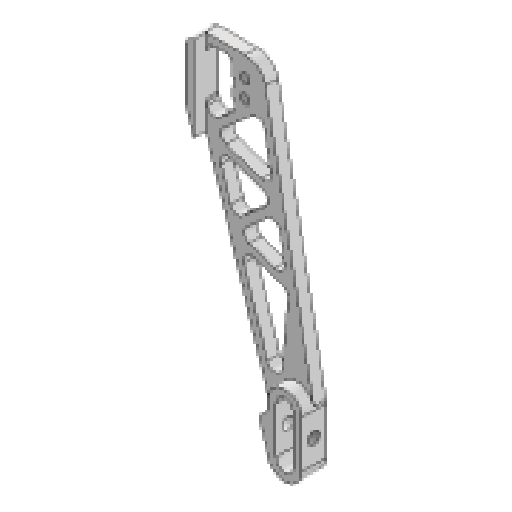
# Autodesk Inventor part: VerticalSlideMiddleTop2.2
Saved by Autodesk Inventor 2023 (Build 270158000, 158)
## iProperties
Created: 2022-10-14
Part Number: VerticalSlideMiddleTop2.2
Material: Generic
Document SubType Name: Modeling
Designer: deli
Density: 1 g/cm^3
Appearance: Default
Mass: 2.31146 g
Surface Area: 29.6295 cm^2
Volume: 2.31146 cm^3
Author: deli
Autodesk Inventor part; units mm, degrees
ref_plane "YZ Plane" through (0, 0, 0) normal (1, 0, 0) x (0, 1, 0)
ref_plane "XZ Plane" through (0, 0, 0) normal (0, 1, 0) x (-1, 0, 0)
ref_plane "XY Plane" through (0, 0, 0) normal (0, 0, 1) x (1, 0, 0)
sketch "Sketch1" plane through (0, 0, 0) normal (0, 0, 1) x (1, 0, 0)
  line L0 (-75.161949, -110.524663) -> (-75.161949, -123.524663)
  line L1 (-75.07064, -124.122072) -> (-53.967918, -191.544158)
  circle A0 centre (-63.161949, -118.274663) radius 1.25
  circle A1 centre (-63.161949, -113.774663) radius 1.25
  arc A2 (-52.161949, -190.274663) -> (-47.661949, -190.274663) centre (-49.911949, -190.274663) ccw
  arc A3 (-47.661949, -178.274663) -> (-52.161949, -178.274663) centre (-49.911949, -178.274663) ccw
  line L2 (-47.661949, -178.274663) -> (-47.661949, -190.274663)
  line L3 (-52.161949, -178.274663) -> (-52.161949, -190.274663)
  line L4 (-45.661949, -178.274663) -> (-45.661949, -190.274663)
  arc A4 (-53.967918, -191.544158) -> (-45.661949, -190.274663) centre (-49.911949, -190.274663) ccw
  arc A5 (-45.661949, -178.274663) -> (-45.736374, -177.482781) centre (-49.911949, -178.274663) ccw
  line L5 (-45.736374, -177.482781) -> (-58.003886, -112.796456)
  line L6 (-73.161949, -108.524663) -> (-63.161949, -108.524663)
  arc A6 (-58.003886, -112.796456) -> (-63.161949, -108.524663) centre (-63.161949, -113.774663) ccw
  arc A7 (-73.161949, -108.524663) -> (-75.161949, -110.524663) centre (-73.161949, -110.524663) ccw
  arc A8 (-75.161949, -123.524663) -> (-75.07064, -124.122072) centre (-73.161949, -123.524663) ccw
  line L7 (-52.161949, -182.774663) -> (-56.161949, -182.774663)
  line L8 (-56.161949, -182.774663) -> (-56.161949, -185.774663)
  line L9 (-56.161949, -185.774663) -> (-52.161949, -185.774663)
  point P0 (0, 0)
  dimension "d2" = 2.5
  dimension "d11" = 2
  dimension "d22" = 12
  dimension "d46" = 2
  dimension "d47" = 4.5
  dimension "d84" = 4
  dimension "d86" = 12
  dimension "d87" = 12
  dimension "d88" = 23
  dimension "d90" = 4
  dimension "d91" = 3
  dimension "d92" = 4.5
  dimension "d94" = 15
  dimension "d96" = 2
  dimension "d147" = 72
  constraints: 20 end point, 16 point on circle, 13 tangent, 9 centre point, 4 equal radius, 4 point on line, 3 perpendicular, 2 coincident, 2 vertical, 1 concentric, 1 horizontal, 1 parallel
  measures "d2" diameter of A0
  measures "d22" distance of A2.centre A3.centre
  measures "d46" radial gap between concentric circles of A4 A2
  measures "d47" distance between parallel lines of L2 L3
  measures "d84" distance edge to line of A1 L6
  measures "d86" distance from line of A1.centre L0
  measures "d87" distance from line of A0.centre L0
  measures "d88" distance between parallel lines of L3 L0
  measures "d90" distance of L7.start L7.end
  measures "d91" distance of L7.end L8.end
  measures "d92" distance from line of L3.start L7
  measures "d94" distance from line of L6 L0.end
  measures "d96" radius of A7
  measures "d147" vertical distance of A2.centre A0.centre
extrude "Extrusion1" add sketch "Sketch1" along normal blind 6.35 contours A7 L6 A6 L5 A5 L4 A4 L1 L9 L3 A2 L2 A3 L7 L8 A8 L0 | L8 L7 L3 L9 L1
thread "Thread2" size "M3x0.5" class "6H" standard "ANSI Metric M Profile" full length
thread "Thread6" size "M3x0.5" class "6H" standard "ANSI Metric M Profile" full length
sketch "Sketch12" plane through (0, 0, 6.35) normal (0, 0, 1) x (1, 0, 0)
  line L0 (-75.161949, -110.524663) -> (-75.161949, -123.524663)
  arc A0 (-75.161949, -123.524663) -> (-75.07064, -124.122072) centre (-73.161949, -123.524663) ccw
  line L1 (-75.07064, -124.122072) -> (-53.967918, -191.544158)
  arc A1 (-53.967918, -191.544158) -> (-45.661949, -190.274663) centre (-49.911949, -190.274663) ccw
  line L2 (-45.661949, -190.274663) -> (-45.661949, -178.274663)
  arc A2 (-45.661949, -178.274663) -> (-45.736374, -177.482781) centre (-49.911949, -178.274663) ccw
  line L3 (-45.736374, -177.482781) -> (-58.003886, -112.796456)
  arc A3 (-58.003886, -112.796456) -> (-63.161949, -108.524663) centre (-63.161949, -113.774663) ccw
  line L4 (-63.161949, -108.524663) -> (-73.161949, -108.524663)
  arc A4 (-73.161949, -108.524663) -> (-75.161949, -110.524663) centre (-73.161949, -110.524663) ccw
  circle A5 centre (-63.161949, -118.274663) radius 1.25
  circle A6 centre (-63.161949, -113.774663) radius 1.25
  line L5 (-47.661949, -178.274663) -> (-47.661949, -190.274663)
  arc A7 (-52.161949, -190.274663) -> (-47.661949, -190.274663) centre (-49.911949, -190.274663) ccw
  line L6 (-52.161949, -190.274663) -> (-52.161949, -178.274663)
  arc A8 (-47.661949, -178.274663) -> (-52.161949, -178.274663) centre (-49.911949, -178.274663) ccw
  line L7 (-73.161949, -123.524663) -> (-73.161949, -110.524663)
  line L8 (-73.161949, -110.524663) -> (-63.161949, -110.524663)
  line L9 (-59.968862, -113.169106) -> (-48.373155, -174.31302)
  line L10 (-54.161949, -184.228661) -> (-73.161949, -123.524663)
  line L11 (-54.161949, -178.274663) -> (-54.161949, -184.228661)
  arc A9 (-65.507157, -116.024663) -> (-60.816741, -116.024663) centre (-63.161949, -118.274663) ccw
  arc A10 (-63.161949, -110.524663) -> (-65.507157, -116.024663) centre (-63.161949, -113.774663) ccw
  arc A11 (-60.816741, -116.024663) -> (-59.968862, -113.169106) centre (-63.161949, -113.774663) ccw
  arc A12 (-48.373155, -174.31302) -> (-54.161949, -178.274663) centre (-49.911949, -178.274663) ccw
  line L12 (-58.885662, -118.8808) -> (-71.275394, -129.552105)
  line L13 (-55.838906, -134.946276) -> (-71.275394, -129.552105)
  line L14 (-71.926138, -127.473015) -> (-64.619282, -121.179603)
  line L15 (-54.930036, -181.774663) -> (-52.161949, -181.774663)
  line L16 (-52.161949, -190.274663) -> (-52.161949, -178.274663)
  line L17 (-70.530854, -131.930874) -> (-55.408607, -137.215235)
  line L18 (-66.017032, -146.352296) -> (-55.408607, -137.215235)
  line L19 (-65.366289, -148.431386) -> (-54.978308, -139.484194)
  line L20 (-65.366289, -148.431386) -> (-52.423802, -152.954046)
  line L21 (-54.610165, -182.796633) -> (-51.993503, -155.223005)
  line L22 (-64.621748, -150.810155) -> (-51.993503, -155.223005)
  point P0 (0, 0)
  point P1 (-54.161949, -181.774663)
  point P2 (-61.040978, -120.737179)
  point P3 (-54.513183, -181.774663)
  dimension "d156" = 2
  dimension "d159" = 2
  dimension "d161" = 2
  dimension "d162" = 2
  dimension "d163" = 2
  dimension "d164" = 2
  dimension "d165" = 2
  dimension "d166" = 2
  dimension "d167" = 60
  dimension "d168" = 60
  dimension "d172" = 2
  dimension "d173" = 3.5
  dimension "d175" = 2
  dimension "d177" = 2
  dimension "d178" = 2
  constraints: 29 end point, 9 point on circle, 7 point on line, 6 parallel, 4 centre point, 2 tangent, 1 perpendicular, 12 other
  measures "d156" distance between parallel lines of L0 L7
  measures "d159" radial gap between concentric circles of A5 A9
  measures "d161" radial gap between concentric circles of A10 A6
  measures "d162" radial gap between concentric circles of A11 A6
  measures "d163" distance between parallel lines of L3 L9
  measures "d164" radial gap between concentric circles of A12 A8
  measures "d165" distance between parallel lines of L6 L11
  measures "d167" angle of L9 L12
  measures "d168" angle of L13 L12
  measures "d172" distance between parallel lines of L12 L14
  measures "d173" distance from line of A2.centre L15
  measures "d175" distance between parallel lines of L13 L17
  measures "d177" distance between parallel lines of L19 L18
  measures "d178" distance between parallel lines of L20 L22
extrude "Extrusion10" cut sketch "Sketch12" against normal blind 10 contours L7 L8 A10 A9 L14 L10 | L12 L9 L13 | L17 L18 L10 | L19 L9 L20 | L22 L21 L15 L10
fillet "Fillet6" radius 2 19 edges at (-73.1619, -110.5247, 3.175) (-63.1619, -110.5247, 3.175) (-65.5072, -116.0247, 3.175) (-64.6193, -121.1796, 3.175) (-71.9261, -127.473, 3.175) (-73.1619, -123.5247, 3.175) (-71.2754, -129.5521, 3.175) (-58.8857, -118.8808, 3.175) (-55.8389, -134.9463, 3.175) (-70.5309, -131.9309, 3.175) (-66.017, -146.3523, 3.175) (-55.4086, -137.2152, 3.175) (-65.3663, -148.4314, 3.175) (-54.9783, -139.4842, 3.175) (-52.4238, -152.954, 3.175) (-51.9935, -155.223, 3.175) (-64.6217, -150.8102, 3.175) (-54.5132, -181.7747, 3.175) (-54.93, -181.7747, 3.175)
sketch "Sketch13" plane through (0, 0, 6.35) normal (0, 0, 1) x (1, 0, 0)
  line L0 (-73.161949, -104.508717) -> (-54.110679, -104.508717)
  line L1 (-54.161949, -181.774663) -> (-73.161949, -181.774663)
  line L2 (-73.161949, -181.774663) -> (-73.161949, -104.508717)
  line L3 (-75.161949, -110.524663) -> (-75.161949, -123.524663)
  arc A0 (-47.661949, -178.274663) -> (-52.161949, -178.274663) centre (-49.911949, -178.274663) ccw
  line L4 (-52.161949, -190.274663) -> (-52.161949, -178.274663)
  line L5 (-56.767657, -143.757101) -> (-60.286305, -148.145679)
  line L6 (-45.736374, -177.482781) -> (-58.003886, -112.796456)
  line L7 (-54.161949, -190.274663) -> (-54.161949, -178.274663)
  arc A1 (-45.661949, -178.274663) -> (-54.161949, -178.274663) centre (-49.911949, -178.274663) ccw
  line L8 (-58.003886, -112.796456) -> (-54.110679, -104.508717)
  point P0 (0, 0)
  point P1 (-45.736374, -177.482781)
  dimension "d134" = 2
  dimension "d135" = 3.5
  dimension "d155" = 2
  constraints: 10 end point, 2 point on circle, 1 centre point, 1 horizontal, 1 parallel, 1 other
  measures "d134" distance between parallel lines of L3 L2
  measures "d135" distance from line of A0.centre L1
  measures "d155" distance between parallel lines of L4 L7
extrude "Extrusion11" cut sketch "Sketch13" against normal blind 3.175
fillet "Fillet11" radius 2 2 edges at (-57.0257, -181.7747, 4.7625) (-54.1619, -181.7747, 4.7625)
sketch "Sketch8" plane through (-52.161949, -190.274663, 0) normal (1, 0, 0) x (0, 0, -1)
  line L0 (0, 0) -> (0, 12) construction
  line L1 (0, 12) -> (-6.35, 12) construction
  line L2 (-6.35, 0) -> (-6.35, 12) construction
  line L3 (0, 0) -> (-6.35, 0) construction
  line L4 (0, 0) -> (-6.35, 0) construction
  line L5 (-6.35, 12) -> (0, 0) construction
  line L6 (-6.35, 0) -> (0, 12) construction
  circle A0 centre (-3.175, 6) radius 1.5
  point P0 (0, 190.274663)
  dimension "d97" = 3
  constraints: 4 end point, 1 centre point, 1 midpoint
  measures "d97" diameter of A0
extrude "Extrusion13" cut sketch "Sketch8" along normal blind 10 and the other way blind 5
thread "Thread7" size "M3x0.5" class "6H" standard "ANSI Metric M Profile" full length
equation "\"d22\" = d17"
equation "\"d17\" = 12"
body "Solid1"
